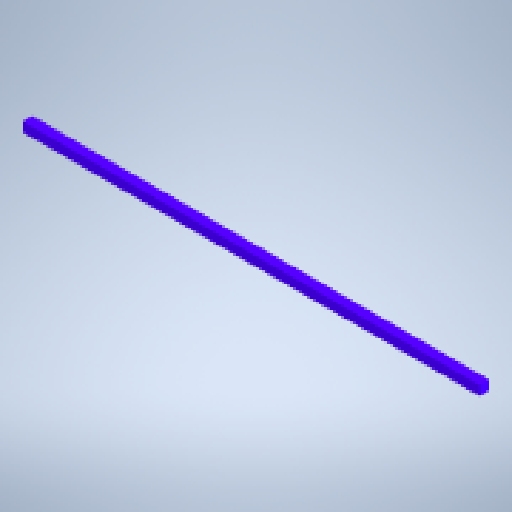
# Autodesk Inventor part: Barra1
Saved by Autodesk Inventor 2024 (Build 280153000, 153)
## iProperties
Created: 2023-07-03
Part Number: Barra1
Material: Genérico
Document SubType Name: Modeling
Designer: sergi
Density: 1 g/cm^3
Appearance: Valor por defecto
Author: sergi
Autodesk Inventor part; units mm, degrees
ref_plane "YZ Plane" through (0, 0, 0) normal (1, 0, 0) x (0, 1, 0)
ref_plane "XZ Plane" through (0, 0, 0) normal (0, 1, 0) x (-1, 0, 0)
ref_plane "XY Plane" through (0, 0, 0) normal (0, 0, 1) x (1, 0, 0)
sketch "Boceto1" plane through (0, 0, 0) normal (0, 1, 0) x (-1, 0, 0)
  line L0 (0, 0) -> (1445, 0)
  line L1 (1445, 0) -> (1445, -30)
  line L2 (1445, -30) -> (0, -30)
  line L3 (0, -30) -> (0, 0)
  line L4 (567, 1400) -> (-30, 1400) projected
  line L5 (567, 0) -> (567, 1400) projected
  line L6 (-30, 0) -> (567, 0) projected
  line L7 (-30, 1400) -> (-30, 0) projected
  line L8 (1470, 0) -> (-30, 0) projected
  line L9 (1470, -597) -> (1470, 0) projected
  line L10 (-30, -597) -> (1470, -597) projected
  line L11 (-30, 0) -> (-30, -597) projected
  line L12 (567, 0) -> (567, -30)
  line L13 (567, 0) -> (537, 0)
  line L14 (537, 0) -> (537, -30)
  line L15 (567, 0) -> (537, -30)
  line L16 (537, 0) -> (537, 1375)
  line L17 (567, 1375) -> (567, 0)
  line L18 (-30, 1400) -> (-30, 1375) projected
  line L19 (567, 1400) -> (-30, 1400) projected
  line L20 (567, 1375) -> (567, 1400) projected
  line L21 (-30, 1375) -> (567, 1375) projected
  line L22 (-30, 1375) -> (-30, -581) projected
  line L23 (-14, 1375) -> (-30, 1375) projected
  line L24 (-14, -581) -> (-14, 1375) projected
  line L25 (-30, -581) -> (-14, -581) projected
  line L26 (567, 1375) -> (537, 1375)
  line L27 (537, 1375) -> (-14, 1375)
  line L28 (537, 1375) -> (537, 1345)
  line L29 (537, 1345) -> (-14, 1345)
  line L30 (-14, 1345) -> (16, 1345)
  line L31 (16, 1345) -> (16, -581)
  line L32 (16, -581) -> (-14, -581)
  line L33 (-14, 1345) -> (-14, -581)
  line L34 (16, -581) -> (1445, -581)
  line L35 (1445, -581) -> (1445, -30)
  line L36 (1445, -30) -> (1415, -30)
  line L37 (1415, -30) -> (1415, -551)
  line L38 (1415, -551) -> (16, -551)
  point P0 (16, -30)
  point P1 (16, 0)
  dimension "d0" = 1445
  dimension "d1" = 30
  dimension "d4" = 30
  dimension "d5" = 30
  dimension "d6" = 30
  dimension "d7" = 30
  dimension "d8" = 521
  constraints: 46 end point, 12 point on line, 8 perpendicular, 3 parallel, 1 collinear, 1 horizontal
  measures "d0" distance of L1.end L2.end
  measures "d1" distance of L0.end L1.end
  measures "d4" distance of L5.start L13.end
  measures "d5" distance of L16.end L28.end
  measures "d6" distance of L29.end L30.end
  measures "d7" distance of L1.end L36.end
  measures "d8" distance of L36.end L37.end
extrude "Extrusión1" add sketch "Boceto1" along normal blind 30 contours L16 L21 L5 L0 | L14 L2 L31 L0 | L0 L15 L14 | L0 L1 L2 L12 | L12 L2 L15 | L31 L2 L3 L0 | L0 L6 L24 L29 L31 | L29 L24 L21 L16 | L3 L2 L31 L32 L24 L6 | L35 L34 L31 L38 L37 L2
